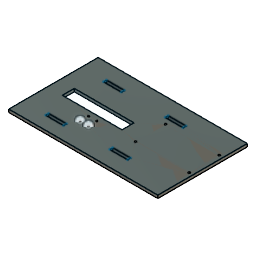
CAD for mechanical car (Autodesk Fusion 360 archive; units mm, degrees)
design "Main Body"
part number: 2026-02-16-11-50-54-130
Autodesk Fusion 360 part; units mm, degrees
(part 1 of 14)
sketch "Sketch1" plane through (0, 0, 0) normal (0, 0, 1) x (1, 0, 0)
  line L0 (0, 0) -> (250, 0)
  line L1 (250, 0) -> (250, 150)
  line L2 (250, 150) -> (0, 150)
  line L3 (0, 150) -> (0, 0)
  line L4 (25, 65) -> (25, 85)
  line L5 (25, 85) -> (125, 85)
  line L6 (125, 85) -> (125, 65)
  line L7 (125, 65) -> (25, 65)
  dimension "d1" = 250
  dimension "d2" = 150
  dimension "d5" = 100
  dimension "d42" = 20
  constraint horizontal L0
  constraint vertical L1
  constraint horizontal L2
  constraint vertical L3
  constraint coincident L0.start L3.end
  constraint perpendicular L5 L6
  constraint perpendicular L4 L7
  measures "d1" distance of L0.start L0.end
  measures "d2" distance of L0.start L2.end
  measures "d5" distance of L4.end L5.end
  measures "d42" distance of L5.end L6.end
extrude "Extrude1" add sketch "Sketch1" along normal blind 5
sketch "Sketch2" plane through (0, 0, 5) normal (0, 0, 1) x (-1, 0, 0)
  line L0 (-125, -85) -> (-125, -65)
  line L1 (-125, -65) -> (-25, -65)
  line L2 (-25, -65) -> (-25, -85)
  line L3 (-25, -85) -> (-125, -85)
  line L4 (0, -150) -> (0, 0)
  line L5 (0, 0) -> (-250, 0)
  line L6 (-250, 0) -> (-250, -150)
  line L7 (-250, -150) -> (0, -150)
  line L8 (-40, -22) -> (-70, -22)
  line L9 (-40, -27) -> (-70, -27)
  line L10 (-70, -27) -> (-70, -22)
  line L11 (-40, -22) -> (-40, -27)
  line L12 (-40, -124) -> (-40, -119)
  line L13 (-40, -124) -> (-70, -124)
  line L14 (-70, -119) -> (-70, -124)
  line L15 (-40, -119) -> (-70, -119)
  line L16 (-143.376, -31) -> (-143.376, -26)
  line L17 (-173.376, -26) -> (-143.376, -26)
  line L18 (-173.376, -26) -> (-173.376, -31)
  line L19 (-173.376, -31) -> (-143.376, -31)
  line L20 (-173.376, -124) -> (-173.376, -119)
  line L21 (-173.376, -119) -> (-143.376, -119)
  line L22 (-143.376, -119) -> (-143.376, -124)
  line L23 (-173.376, -124) -> (-143.376, -124)
  dimension "d10" = 30
  dimension "d34" = 26
  dimension "d35" = 5
  dimension "d36" = 26
  dimension "d37" = 5
  dimension "d38" = 26
  dimension "d39" = 5
  dimension "d40" = 5
  dimension "d41" = 22
  constraint perpendicular L8 L10
  constraint perpendicular L9 L11
  measures "d10" distance of L8.start L8.end
  measures "d34" distance of L7 L13
  measures "d35" distance of L13 L15
  measures "d36" distance of L7 L23
  measures "d37" distance of L21 L23
  measures "d38" distance of L5 L17
  measures "d39" distance of L17 L19
  measures "d40" distance of L8 L9
  measures "d41" distance of L5 L8
extrude "Extrude2" cut sketch "Sketch2" against normal blind 10 contours L8 L9 L10 L11 | L12 L13 L14 L15 | L16 L17 L18 L19 | L20 L21 L22 L23
sketch "Sketch3" plane through (0, 0, 5) normal (0, 0, 1) x (-1, 0, 0)
  line L0 (-143.376, -31) -> (-173.376, -31)
  line L1 (-173.376, -31) -> (-173.376, -26)
  line L2 (-173.376, -26) -> (-143.376, -26)
  line L3 (-143.376, -26) -> (-143.376, -31)
  line L4 (-143.376, -124) -> (-173.376, -124)
  line L5 (-173.376, -124) -> (-173.376, -119)
  line L6 (-173.376, -119) -> (-143.376, -119)
  line L7 (-143.376, -119) -> (-143.376, -124)
  line L8 (-70, -27) -> (-70, -22)
  line L9 (-70, -22) -> (-40, -22)
  line L10 (-40, -22) -> (-40, -27)
  line L11 (-40, -27) -> (-70, -27)
  line L12 (-70, -119) -> (-40, -119)
  line L13 (-40, -119) -> (-40, -124)
  line L14 (-40, -124) -> (-70, -124)
  line L15 (-70, -124) -> (-70, -119)
  line L16 (-125, -85) -> (-125, -65)
  line L17 (-125, -65) -> (-25, -65)
  line L18 (-25, -65) -> (-25, -85)
  line L19 (-25, -85) -> (-125, -85)
  line L20 (0, -150) -> (0, 0)
  line L21 (0, 0) -> (-250, 0)
  line L22 (-250, 0) -> (-250, -150)
  line L23 (-250, -150) -> (0, -150)
  circle A0 centre (-91.302, -56.5) radius 1.75
  circle A1 centre (-91.302, -42.5) radius 1.75
  circle A2 centre (-77.302, -56.5) radius 1.75
  circle A3 centre (-77.302, -42.5) radius 1.75
  line L24 (-245.676, -150) -> (-245.676, -100) construction
  line L25 (-245.676, 0) -> (-245.676, -50) construction
  point P0 (-245.676, -100)
  point P1 (-245.676, -50)
  dimension "d21" = 3.5
  dimension "d43" = 4.324
  dimension "d44" = 4.324
  constraint coincident L23 L24.start
  constraint perpendicular L23 L24
  constraint coincident L21 L25.start
  constraint perpendicular L21 L25
  constraint coincident P0 L24.end
  constraint coincident P1 L25.end
  measures "d21" diameter of A0
  measures "d43" distance of L22 L24
  measures "d44" distance of L22 L25
extrude "Extrude3" cut sketch "Sketch3" against normal blind 5 contours A0 | A1 | A2 | A3
thread "Thread1" "ISO Metric profile 3.5 M3.5x0.6 M3.5x0.6 6H" major diameter 3.5995 minor diameter 2.93 pitch 0.6 angle 60 resizes the face on face at (75.6894, 57.1798, 3.3333)
thread "Thread2" "ISO Metric profile 3.5 M3.5x0.6 M3.5x0.6 6H" major diameter 3.5995 minor diameter 2.93 pitch 0.6 angle 60 resizes the face on face at (89.6894, 57.1798, 3.3333)
thread "Thread3" "ISO Metric profile 3.5 M3.5x0.6 M3.5x0.6 6H" major diameter 3.5995 minor diameter 2.93 pitch 0.6 angle 60 resizes the face on face at (75.6894, 43.1798, 3.3333)
thread "Thread4" "ISO Metric profile 3.5 M3.5x0.6 M3.5x0.6 6H" major diameter 3.5995 minor diameter 2.93 pitch 0.6 angle 60 resizes the face on face at (89.6894, 43.1798, 3.3333)
sketch "Sketch4" plane through (0, 0, 5) normal (0, 0, 1) x (-1, 0, 0)
  circle A0 centre (-91.302, -56.5) radius 1.465
  circle A1 centre (-91.302, -42.5) radius 1.465
  circle A2 centre (-77.302, -56.5) radius 1.465
  circle A3 centre (-77.302, -42.5) radius 1.465
  line L0 (-143.376, -31) -> (-173.376, -31)
  line L1 (-173.376, -31) -> (-173.376, -26)
  line L2 (-173.376, -26) -> (-143.376, -26)
  line L3 (-143.376, -26) -> (-143.376, -31)
  line L4 (-143.376, -124) -> (-173.376, -124)
  line L5 (-173.376, -124) -> (-173.376, -119)
  line L6 (-173.376, -119) -> (-143.376, -119)
  line L7 (-143.376, -119) -> (-143.376, -124)
  line L8 (-70, -27) -> (-70, -22)
  line L9 (-70, -22) -> (-40, -22)
  line L10 (-40, -22) -> (-40, -27)
  line L11 (-40, -27) -> (-70, -27)
  line L12 (-70, -119) -> (-40, -119)
  line L13 (-40, -119) -> (-40, -124)
  line L14 (-40, -124) -> (-70, -124)
  line L15 (-70, -124) -> (-70, -119)
  line L16 (-125, -85) -> (-125, -65)
  line L17 (-125, -65) -> (-25, -65)
  line L18 (-25, -65) -> (-25, -85)
  line L19 (-25, -85) -> (-125, -85)
  line L20 (0, -150) -> (0, 0)
  line L21 (0, 0) -> (-250, 0)
  line L22 (-250, 0) -> (-250, -150)
  line L23 (-250, -150) -> (0, -150)
sketch "Sketch5" plane through (0, 0, 5) normal (0, 0, 1) x (-1, 0, 0)
  circle A0 centre (-91.302, -56.5) radius 1.465
  circle A1 centre (-91.302, -42.5) radius 1.465
  circle A2 centre (-77.302, -56.5) radius 1.465
  circle A3 centre (-77.302, -42.5) radius 1.465
  line L0 (-143.376, -31) -> (-173.376, -31)
  line L1 (-173.376, -31) -> (-173.376, -26)
  line L2 (-173.376, -26) -> (-143.376, -26)
  line L3 (-143.376, -26) -> (-143.376, -31)
  line L4 (-143.376, -124) -> (-173.376, -124)
  line L5 (-173.376, -124) -> (-173.376, -119)
  line L6 (-173.376, -119) -> (-143.376, -119)
  line L7 (-143.376, -119) -> (-143.376, -124)
  line L8 (-70, -27) -> (-70, -22)
  line L9 (-70, -22) -> (-40, -22)
  line L10 (-40, -22) -> (-40, -27)
  line L11 (-40, -27) -> (-70, -27)
  line L12 (-70, -119) -> (-40, -119)
  line L13 (-40, -119) -> (-40, -124)
  line L14 (-40, -124) -> (-70, -124)
  line L15 (-70, -124) -> (-70, -119)
  line L16 (-125, -85) -> (-125, -65)
  line L17 (-125, -65) -> (-25, -65)
  line L18 (-25, -65) -> (-25, -85)
  line L19 (-25, -85) -> (-125, -85)
  line L20 (0, -150) -> (0, 0)
  line L21 (0, 0) -> (-250, 0)
  line L22 (-250, 0) -> (-250, -150)
  line L23 (-250, -150) -> (0, -150)
  line L24 (-244.9961, -70.043) -> (-245.7331, -70.043) construction
  line L25 (-245.7331, -70.043) -> (-240.4599, -70.043) construction
  circle A4 centre (-243.5877, -109.541) radius 2
  circle A5 centre (-153.5877, -109.541) radius 2
  line L26 (-153.5877, -119) -> (-153.5877, -109.541)
  line L27 (-153.5877, -109.541) -> (-243.5877, -109.541)
  line L28 (-153.5802, -70.983) -> (-153.5877, -59.041)
  circle A6 centre (-153.5877, -59.041) radius 2
  line L29 (-153.5877, -59.041) -> (-243.5877, -59.0974)
  circle A7 centre (-243.5877, -59.0974) radius 2
  line L30 (-153.5877, -109.541) -> (-153.5877, -59.041)
  point P0 (-243.5877, -109.541)
  point P1 (-153.5877, -109.541)
  dimension "d46" = 4
  dimension "d47" = 4
  dimension "d52" = 9.459
  dimension "d53" = 90
  dimension "d56" = 11.942
  dimension "d57" = 4
  dimension "d58" = 90
  dimension "d59" = 4
  dimension "d62" = 50.5
  constraint coincident P0 A4.centre
  constraint coincident P1 A5.centre
  constraint coincident L6 L26.start
  constraint perpendicular L6 L26
  constraint perpendicular L26 L27
  constraint coincident L28.end A6.centre
  constraint perpendicular L28 L29
  constraint coincident L29.end A7.centre
  constraint perpendicular L27 L30
  measures "d46" diameter of A4
  measures "d47" diameter of A5
  measures "d52" distance of L26.start P1
  measures "d53" distance of P1 P0
  measures "d56" distance of L28.start L28.end
  measures "d57" diameter of A6
  measures "d58" distance of L28.end L29.end
  measures "d59" diameter of A7
  measures "d62" distance of P1 L28.end
hole "Hole1" at (243.5877, 109.541, 5) at (153.5877, 109.541, 5) at (153.5877, 59.041, 5) at (243.5877, 59.0974, 5) direction (0, 0, -1) diameter 3.332 depth 15 tip angle 180
thread "Thread5" "ISO Metric profile 4.0 M4x0.7 M4x0.7 6H" major diameter 4.1095 minor diameter 3.332 pitch 0.7 angle 60 resizes the face on face at (152.5818, 108.213, 3.3333) on face at (242.5818, 57.7694, 3.3333) on face at (242.5818, 108.213, 3.3333) on face at (152.5818, 57.713, 3.3333)
sketch "Sketch6" plane through (0, 0, 5) normal (0, 0, 1) x (-1, 0, 0)
  point P0 (-77.3, -42.5)
  point P1 (-91.3, -42.5)
equation "d43 = 2.9 mm + 1.424 mm"
equation "d44 = 2.9 mm + 1.424 mm"

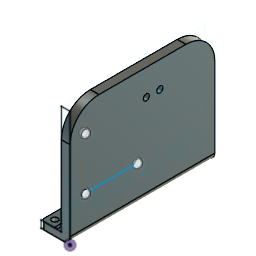
design "bracket left stopping mechanism"
part number: 2026-03-17-00-30-14-356
Autodesk Fusion 360 part; units mm, degrees
sketch "Sketch1" plane through (0, 0, 0) normal (0, 1, 0) x (1, 0, 0)
  line L0 (-20, 0) -> (0, 0)
  line L1 (0, 0) -> (0, -80)
  line L2 (0, -80) -> (-6, -80)
  line L3 (-6, -80) -> (-6, -5)
  line L4 (-6, -5) -> (-20, -5)
  line L5 (-20, -5) -> (-20, 0)
  dimension "d6" = 80
  dimension "d7" = 6
  dimension "d8" = 75
  dimension "d41" = 5
  dimension "d42" = 14
  constraint coincident L0.end L1.start
  constraint horizontal L0
  constraint perpendicular L0 L1
  constraint perpendicular L1 L2
  constraint perpendicular L0 L3
  constraint perpendicular L3 L4
  constraint perpendicular L0 L5
  measures "d6" distance of L0.end L1.end
  measures "d7" distance of L1.end L2.end
  measures "d8" distance of L2.end L3.end
  measures "d41" distance of L0.start L4.end
  measures "d42" distance of L3.end L4.end
extrude "Extrude1" add sketch "Sketch1" along normal blind 100
sketch "Sketch2" plane through (-6, 0, 0) normal (-1, 0, 0) x (0, -1, 0)
  line L0 (0, 5) -> (0, 80)
  line L1 (0, 80) -> (-100, 80)
  line L2 (-100, 80) -> (-100, 5)
  line L3 (-100, 5) -> (0, 5)
sketch "Sketch3" plane through (-6, 0, 0) normal (-1, 0, 0) x (0, -1, 0)
  circle A0 centre (-62, 62) radius 2.1
  line L0 (0, 80) -> (-100, 80)
  line L1 (0, 5) -> (-100, 5)
  line L2 (0, 5) -> (0, 80)
  line L3 (0, 0) -> (0, 80)
  dimension "d12" = 4.2
  dimension "d57" = 62
  measures "d12" diameter of A0
  measures "d57" distance of A0.centre L3
sketch "Sketch4" plane through (-6, 0, 0) normal (-1, 0, 0) x (0, -1, 0)
sketch "Sketch5" plane through (-6, 0, 0) normal (-1, 0, 0) x (0, -1, 0)
extrude "Extrude2" cut sketch "Sketch3" against normal blind 6
fillet "Fillet1" radius 20 1 edges at (-3, 100, 80)
fillet "Fillet2" radius 20 1 edges at (-3, 0, 80)
fillet "Fillet3" radius 5 1 edges at (-6, 50, 5)
sketch "Sketch7" plane through (0, 0, 5) normal (0, 0, 1) x (-1, 0, 0)
  line L0 (11, 0) -> (11, -100)
  line L1 (11, -100) -> (20, -100)
  line L2 (20, -100) -> (20, 0)
  line L3 (20, 0) -> (11, 0)
sketch "Sketch8" plane through (0, 0, 5) normal (0, 0, 1) x (-1, 0, 0)
  circle A0 centre (15.5, -5) radius 2.1
  dimension "d28" = 4.2
  measures "d28" diameter of A0
extrude "Extrude4" cut sketch "Sketch8" against normal blind 5
sketch "Sketch9" plane through (0, 0, 5) normal (0, 0, 1) x (-1, 0, 0)
sketch "Sketch10" plane through (0, 0, 5) normal (0, 0, 1) x (-1, 0, 0)
  circle A0 centre (15, -95) radius 2.1
  dimension "d32" = 4.2
  measures "d32" diameter of A0
extrude "Extrude5" cut sketch "Sketch10" against normal blind 5
fillet "Fillet4" radius 2 1 edges at (-20, 0, 2.5)
fillet "Fillet5" radius 2 1 edges at (-20, 100, 2.5)
fillet "Fillet6" radius 5 1 edges at (0, 50, 0)
sketch "Sketch11" plane through (0, 0, 0) normal (1, 0, 0) x (0, 1, 0)
  line L0 (0, 5) -> (100, 5)
  line L1 (100, 5) -> (100, 60)
  arc A0 (100, 60) -> (80, 80) centre (80, 60) ccw
  line L2 (80, 80) -> (20, 80)
  arc A1 (20, 80) -> (0, 60) centre (20, 60) ccw
  line L3 (0, 60) -> (0, 5)
  circle A2 centre (62, 62) radius 2.1
sketch "Sketch12" plane through (0, 0, 0) normal (1, 0, 0) x (0, 1, 0)
sketch "Sketch13" plane through (0, 0, 0) normal (1, 0, 0) x (0, 1, 0)
sketch "Sketch14" plane through (0, 0, 0) normal (1, 0, 0) x (0, 1, 0)
sketch "Sketch15" plane through (0, 0, 0) normal (1, 0, 0) x (0, 1, 0)
sketch "Sketch17" plane through (0, 0, 0) normal (1, 0, 0) x (0, 1, 0)
  circle A0 centre (10, 62) radius 2.1
  dimension "d54" = 4.2
  measures "d54" diameter of A0
extrude "Extrude6" cut sketch "Sketch17" against normal blind 6
sketch "Sketch18" plane through (0, 0, 0) normal (1, 0, 0) x (0, 1, 0)
sketch "Sketch19" plane through (0, 0, 0) normal (1, 0, 0) x (0, 1, 0)
sketch "Sketch20" plane through (0, 0, 0) normal (1, 0, 0) x (0, 1, 0)
  circle A0 centre (10, 26) radius 2.1
  dimension "d59" = 4.2
  measures "d59" diameter of A0
extrude "Extrude7" cut sketch "Sketch20" against normal blind 6
sketch "Sketch21" plane through (0, 0, 0) normal (1, 0, 0) x (0, 1, 0)
sketch "Sketch22" plane through (0, 0, 0) normal (1, 0, 0) x (0, 1, 0)
  point P0 (10, 62)
sketch "Sketch23" plane through (0, 0, 0) normal (1, 0, 0) x (0, 1, 0)
sketch "Sketch24" plane through (0, 0, 0) normal (1, 0, 0) x (0, 1, 0)
  line L0 (10, 26) -> (46, 26)
  dimension "d62" = 36
  constraint horizontal L0
  measures "d62" distance of L0.start L0.end
sketch "Sketch25" plane through (0, 0, 0) normal (1, 0, 0) x (0, 1, 0)
  line L0 (10, 62) -> (52.686, 62)
  circle A0 centre (52.686, 62) radius 2.1
  dimension "d63" = 42.686
  dimension "d64" = 4.2
  constraint horizontal L0
  constraint coincident L0.end A0.centre
  measures "d63" distance of L0.start L0.end
  measures "d64" diameter of A0
extrude "Extrude8" cut sketch "Sketch25" against normal blind 6

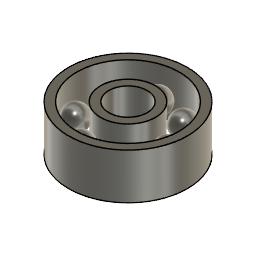
design "Bearing 4.2x13"
part number: 2026-09-12-01-25-43-170
Autodesk Fusion 360 part; units mm, degrees
sketch "Sketch1" plane through (0, 0, 0) normal (0, 1, 0) x (1, 0, 0)
  line L0 (2.1, -2.5) -> (3, -2.5)
  line L1 (3, -2.5) -> (3, 2.5)
  line L2 (3, 2.5) -> (2.1, 2.5)
  line L3 (2.1, 2.5) -> (2.1, -2.5)
  line L4 (5.6, -2.5) -> (6.5, -2.5)
  line L5 (6.5, -2.5) -> (6.5, 2.5)
  line L6 (6.5, 2.5) -> (5.6, 2.5)
  line L7 (5.6, 2.5) -> (5.6, -2.5)
  line L8 (0, -10) -> (0, 10) construction
revolve "Revolve1" add sketch "Sketch1" angle 360 about axis through (0, 0, 10) along (0, 0, -1) contours L0 L1 L2 L3 makes body 1
revolve "Revolve2" add sketch "Sketch1" angle 360 about axis through (0, 0, 10) along (0, 0, -1) separate body contours L4 L5 L6 L7 makes body 2
sketch "Sketch2" plane through (0, 0, 0) normal (0, 1, 0) x (1, 0, 0)
  line L0 (4.3, -10) -> (4.3, 10) construction
  arc A0 (4.3, -1.3) -> (4.3, 1.3) centre (4.3, 0) ccw
  line L1 (4.3, 1.3) -> (4.3, -1.3)
revolve "Revolve3" add sketch "Sketch2" angle 360 about axis through (4.3, 0, 10) along (0, 0, -1) separate body makes body 3
pattern_circular "C-Pattern2" count 7 over 360 about axis through (0, 0, 1.75) along (0, 0, 1) of bodies 3 makes body 4 at (3.6897, 4.1339, 0.2766) makes body 5 at (-0.9315, 5.4622, 0.2766) makes body 6 at (-4.8513, 2.6773, 0.2766) makes body 7 at (-5.1179, -2.1236, 0.2766) makes body 8 at (-1.5307, -5.3254, 0.2766) makes body 9 at (3.2092, -4.5171, 0.2766)
named bodies: "Inner Race", "Outer Race", "Ball", "Ball (1)", "Ball (2)", "Ball (3)", "Ball (4)", "Ball (5)", "Ball (6)"

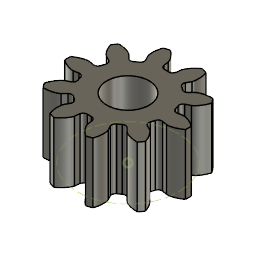
design "Smaller 10 Tooth Gear"
description: Spur Gear; Module: 1.0; Num Teeth: 10; Pressure Angle: 20.0; Backlash: 0.00 mm
part number: 2026-09-03-00-38-16-628
Autodesk Fusion 360 part; units mm, degrees
sketch "Base Circle" plane through (0, 0, 0) normal (0, 0, 1) x (1, 0, 0)
  circle A0 centre (0, 0) radius 3.843
  circle A1 centre (0, 0) radius 2.1
extrude "Extrude1" add sketch "Base Circle" along normal blind 6
sketch "Gear Tooth" plane through (0, 0, 0) normal (0, 0, 1) x (1, 0, 0)
  spline S0 degree 5 poles (4.6291, -0.8041) (4.6329, -0.8047) (4.6405, -0.8059) (4.6519, -0.8073) (4.6672, -0.8084) (4.6864, -0.8088) (4.7057, -0.8085) (4.7251, -0.8077) (4.7445, -0.8066) (4.7639, -0.8054) (4.7834, -0.804) (4.8029, -0.8024) (4.8224, -0.8004) (4.842, -0.7981) (4.8616, -0.7955) (4.8812, -0.7924) (4.9009, -0.7891) (4.9205, -0.7856) (4.9402, -0.7818) (4.9599, -0.7778) (4.9796, -0.7737) (4.9993, -0.7693) (5.019, -0.7646) (5.0388, -0.7598) (5.0585, -0.7547) (5.0783, -0.7493) (5.098, -0.7438) (5.1178, -0.738) (5.1375, -0.7321) (5.1573, -0.7259) (5.177, -0.7196) (5.1968, -0.7131) (5.2165, -0.7063) (5.2363, -0.6994) (5.256, -0.6923) (5.2757, -0.685) (5.2955, -0.6775) (5.3152, -0.6698) (5.3349, -0.6619) (5.3546, -0.6538) (5.3743, -0.6456) (5.394, -0.6372) (5.4136, -0.6286) (5.4333, -0.6198) (5.4529, -0.6109) (5.4725, -0.6018) (5.4921, -0.5925) (5.5117, -0.583) (5.5312, -0.5734) (5.5508, -0.5636) (5.5703, -0.5536) (5.5898, -0.5435) (5.6093, -0.5332) (5.6287, -0.5228) (5.6482, -0.5121) (5.6676, -0.5013) (5.6869, -0.4904) (5.7063, -0.4793) (5.7256, -0.468) (5.7449, -0.4566) (5.7642, -0.445) (5.7834, -0.4332) (5.8026, -0.4213) (5.8218, -0.4093) (5.8409, -0.397) (5.86, -0.3847) (5.8791, -0.3721) (5.8982, -0.3595) (5.9172, -0.3466) (5.9361, -0.3336) (5.9551, -0.3205) (5.9702, -0.3099) (5.9815, -0.3018) (5.989, -0.2964) (5.9928, -0.2937) knots 0 0 0 0 0 0 0.01428571 0.02857143 0.04285714 0.05714286 0.07142857 0.08571429 0.1 0.11428571 0.12857143 0.14285714 0.15714286 0.17142857 0.18571429 0.2 0.21428571 0.22857143 0.24285714 0.25714286 0.27142857 0.28571429 0.3 0.31428571 0.32857143 0.34285714 0.35714286 0.37142857 0.38571429 0.4 0.41428571 0.42857143 0.44285714 0.45714286 0.47142857 0.48571429 0.5 0.51428571 0.52857143 0.54285714 0.55714286 0.57142857 0.58571429 0.6 0.61428571 0.62857143 0.64285714 0.65714286 0.67142857 0.68571429 0.7 0.71428571 0.72857143 0.74285714 0.75714286 0.77142857 0.78571429 0.8 0.81428571 0.82857143 0.84285714 0.85714286 0.87142857 0.88571429 0.9 0.91428571 0.92857143 0.94285714 0.95714286 0.97142857 0.98571429 1 1 1 1 1 1
  spline S1 degree 5 poles (4.6291, 0.8041) (4.6329, 0.8047) (4.6405, 0.8059) (4.6519, 0.8073) (4.6672, 0.8084) (4.6864, 0.8088) (4.7057, 0.8085) (4.7251, 0.8077) (4.7445, 0.8066) (4.7639, 0.8054) (4.7834, 0.804) (4.8029, 0.8024) (4.8224, 0.8004) (4.842, 0.7981) (4.8616, 0.7955) (4.8812, 0.7924) (4.9009, 0.7891) (4.9205, 0.7856) (4.9402, 0.7818) (4.9599, 0.7778) (4.9796, 0.7737) (4.9993, 0.7693) (5.019, 0.7646) (5.0388, 0.7598) (5.0585, 0.7547) (5.0783, 0.7493) (5.098, 0.7438) (5.1178, 0.738) (5.1375, 0.7321) (5.1573, 0.7259) (5.177, 0.7196) (5.1968, 0.7131) (5.2165, 0.7063) (5.2363, 0.6994) (5.256, 0.6923) (5.2757, 0.685) (5.2955, 0.6775) (5.3152, 0.6698) (5.3349, 0.6619) (5.3546, 0.6538) (5.3743, 0.6456) (5.394, 0.6372) (5.4136, 0.6286) (5.4333, 0.6198) (5.4529, 0.6109) (5.4725, 0.6018) (5.4921, 0.5925) (5.5117, 0.583) (5.5312, 0.5734) (5.5508, 0.5636) (5.5703, 0.5536) (5.5898, 0.5435) (5.6093, 0.5332) (5.6287, 0.5228) (5.6482, 0.5121) (5.6676, 0.5013) (5.6869, 0.4904) (5.7063, 0.4793) (5.7256, 0.468) (5.7449, 0.4566) (5.7642, 0.445) (5.7834, 0.4332) (5.8026, 0.4213) (5.8218, 0.4093) (5.8409, 0.397) (5.86, 0.3847) (5.8791, 0.3721) (5.8982, 0.3595) (5.9172, 0.3466) (5.9361, 0.3336) (5.9551, 0.3205) (5.9702, 0.3099) (5.9815, 0.3018) (5.989, 0.2964) (5.9928, 0.2937) knots 0 0 0 0 0 0 0.01428571 0.02857143 0.04285714 0.05714286 0.07142857 0.08571429 0.1 0.11428571 0.12857143 0.14285714 0.15714286 0.17142857 0.18571429 0.2 0.21428571 0.22857143 0.24285714 0.25714286 0.27142857 0.28571429 0.3 0.31428571 0.32857143 0.34285714 0.35714286 0.37142857 0.38571429 0.4 0.41428571 0.42857143 0.44285714 0.45714286 0.47142857 0.48571429 0.5 0.51428571 0.52857143 0.54285714 0.55714286 0.57142857 0.58571429 0.6 0.61428571 0.62857143 0.64285714 0.65714286 0.67142857 0.68571429 0.7 0.71428571 0.72857143 0.74285714 0.75714286 0.77142857 0.78571429 0.8 0.81428571 0.82857143 0.84285714 0.85714286 0.87142857 0.88571429 0.9 0.91428571 0.92857143 0.94285714 0.95714286 0.97142857 0.98571429 1 1 1 1 1 1
  arc A0 (5.9928, -0.2937) -> (5.9928, 0.2937) centre (0, 0) ccw
  line L0 (3.7765, -0.656) -> (4.6291, -0.8041)
  line L1 (3.7765, 0.656) -> (4.6291, 0.8041)
  line L2 (3.7765, -0.656) -> (3.7765, 0.656)
  point P0 (4.7229, -0.8077)
  point P1 (4.8183, -0.8008)
  point P2 (4.9148, -0.7866)
  point P3 (5.0121, -0.7662)
  point P4 (5.11, -0.7403)
  point P5 (5.2082, -0.7091)
  point P6 (5.3067, -0.673)
  point P7 (5.4054, -0.6322)
  point P8 (5.504, -0.5867)
  point P9 (5.6025, -0.5368)
  point P10 (5.7007, -0.4824)
  point P11 (5.7986, -0.4238)
  point P12 (5.896, -0.3609)
  point P13 (4.7229, 0.8077)
  point P14 (4.8183, 0.8008)
  point P15 (4.9148, 0.7866)
  point P16 (5.0121, 0.7662)
  point P17 (5.11, 0.7403)
  point P18 (5.2082, 0.7091)
  point P19 (5.3067, 0.673)
  point P20 (5.4054, 0.6322)
  point P21 (5.504, 0.5867)
  point P22 (5.6025, 0.5368)
  point P23 (5.7007, 0.4824)
  point P24 (5.7986, 0.4238)
  point P25 (5.896, 0.3609)
extrude "Extrude2" add sketch "Gear Tooth" along normal blind 6
fillet "Fillet1" radius 0.38 2 edges at (3.7863, -0.6577, 3) (3.7863, 0.6577, 3)
pattern_circular "C-Pattern1" count 10 over 360 about axis through (0, 0, 0) along (0, 0, 1) of "Extrude2", "Fillet1"
sketch "Diametrial Pitch Circle" plane through (0, 0, 0) normal (0, 0, 1) x (1, 0, 0)
  circle A0 centre (0, 0) radius 5 construction
named bodies: "Spur Gear (10 teeth)"

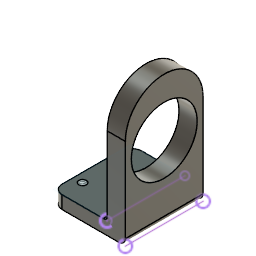
design "motor mount"
part number: 2026-09-09-23-18-51-643
Autodesk Fusion 360 part; units mm, degrees
sketch "Sketch1" plane through (0, 0, 0) normal (0, 1, 0) x (1, 0, 0)
  line L0 (0, 0) -> (0, -50)
  line L1 (0, -50) -> (-7.035, -50)
  line L2 (-7.035, -50) -> (-7.035, -5)
  line L3 (-7.035, -5) -> (-27.965, -5)
  line L4 (-27.965, -5) -> (-27.965, 0)
  line L5 (-27.965, 0) -> (0, 0)
  dimension "d1" = 50
  dimension "d2" = 7.035
  dimension "d3" = 45
  dimension "d4" = 20.93
  constraint coincident L0.start L5.end
  constraint vertical L0
  constraint perpendicular L0 L1
  constraint perpendicular L1 L2
  constraint perpendicular L2 L3
  constraint perpendicular L3 L4
  constraint perpendicular L0 L5
  measures "d1" distance of L0.start L0.end
  measures "d2" distance of L0.end L1.end
  measures "d3" distance of L1.end L2.end
  measures "d4" distance of L2.end L3.end
extrude "Extrude1" add sketch "Sketch1" along normal blind 30
sketch "Sketch2" plane through (0, 0, 0) normal (1, 0, 0) x (0, 1, 0)
sketch "Sketch4" plane through (0, 0, 0) normal (1, 0, 0) x (0, 1, 0)
  line L0 (0, 0) -> (30, 0)
  dimension "d9" = 30
  measures "d9" distance of L0.start L0.end
sketch "Sketch5" plane through (0, 0, 0) normal (1, 0, 0) x (0, 1, 0)
sketch "Sketch6" plane through (0, 0, 0) normal (1, 0, 0) x (0, 1, 0)
fillet "Fillet3" radius 2.5 1 edges at (0, 15, 0)
sketch "Sketch8" plane through (0, 0, 5) normal (0, 0, 1) x (-1, 0, 0)
  line L0 (27.965, 0) -> (7.035, 0)
  line L1 (7.035, 0) -> (7.035, -30)
  line L2 (7.035, -30) -> (27.965, -30)
  line L3 (27.965, -30) -> (27.965, 0)
sketch "Sketch9" plane through (0, 0, 5) normal (0, 0, 1) x (-1, 0, 0)
  circle A0 centre (10.4981, -26.535) radius 1.465
  line L0 (7.035, -30) -> (27.965, -30)
  dimension "d20" = 2.93
  dimension "d24" = 3.465
  measures "d20" diameter of A0
  measures "d24" distance of A0.centre L0
sketch "Sketch10" plane through (0, 0, 5) normal (0, 0, 1) x (1, 0, 0)
sketch "Sketch11" plane through (0, 0, 5) normal (0, 0, 1) x (1, 0, 0)
sketch "Sketch12" plane through (0, 0, 5) normal (0, 0, 1) x (-1, 0, 0)
sketch "Sketch13" plane through (0, 0, 5) normal (0, 0, 1) x (-1, 0, 0)
sketch "Sketch14" plane through (0, 0, 5) normal (0, 0, 1) x (-1, 0, 0)
  line L0 (7.035, 0) -> (7.035, -30)
sketch "Sketch21" plane through (0, 0, 5) normal (0, 0, 1) x (-1, 0, 0)
sketch "Sketch22" plane through (0, 0, 5) normal (0, 0, 1) x (-1, 0, 0)
sketch "Sketch23" plane through (0, 0, 5) normal (0, 0, 1) x (-1, 0, 0)
sketch "Sketch25" plane through (0, 0, 5) normal (0, 0, 1) x (-1, 0, 0)
fillet "Fillet4" radius 4.5 1 edges at (-27.965, 30, 2.5)
fillet "Fillet5" radius 3.5 1 edges at (-27.965, 0, 2.5)
fillet "Fillet6" radius 1.5 tangency weight 1.75178 1 edges at (-7.035, 15, 5)
sketch "Sketch32" plane through (0, 0, 5) normal (0, 0, 1) x (-1, 0, 0)
sketch "Sketch33" plane through (0, 0, 5) normal (0, 0, 1) x (1, 0, 0)
sketch "Sketch40" plane through (0, 0, 5) normal (0, 0, 1) x (-1, 0, 0)
sketch "Sketch44" plane through (0, 0, 5) normal (0, 0, 1) x (-1, 0, 0)
  circle A0 centre (10.5, -8) radius 1.465
  dimension "d82" = 2.93
  measures "d82" diameter of A0
sketch "Sketch46" plane through (0, 0, 5) normal (0, 0, 1) x (-1, 0, 0)
  circle A0 centre (10.5, -22) radius 1.465
  dimension "d84" = 2.93
  measures "d84" diameter of A0
sketch "Sketch48" plane through (0, 0, 5) normal (0, 0, 1) x (-1, 0, 0)
  circle A0 centre (24.5, -22) radius 1.465
  dimension "d86" = 2.93
  measures "d86" diameter of A0
sketch "Sketch49" plane through (0, 0, 5) normal (0, 0, 1) x (-1, 0, 0)
  circle A0 centre (24.5, -8) radius 1.465
  dimension "d87" = 2.93
  measures "d87" diameter of A0
extrude "Extrude8" cut sketch "Sketch49" against normal blind 10
extrude "Extrude9" cut sketch "Sketch44" against normal blind 10
extrude "Extrude10" cut sketch "Sketch46" against normal blind 10
extrude "Extrude11" cut sketch "Sketch48" against normal blind 10
thread "Thread5" "ISO Metric profile 3.5 M3.5x0.6 M3.5x0.6 6H" major diameter 3.5995 minor diameter 2.93 pitch 0.6 angle 60 resizes the face on face at (-25.9577, 8.1459, 3.3333)
thread "Thread6" "ISO Metric profile 3.5 M3.5x0.6 M3.5x0.6 6H" major diameter 3.5995 minor diameter 2.93 pitch 0.6 angle 60 resizes the face on face at (-11.9577, 8.1459, 3.3333)
thread "Thread7" "ISO Metric profile 3.5 M3.5x0.6 M3.5x0.6 6H" major diameter 3.5995 minor diameter 2.93 pitch 0.6 angle 60 resizes the face on face at (-11.9577, 22.1459, 3.3333)
thread "Thread8" "ISO Metric profile 3.5 M3.5x0.6 M3.5x0.6 6H" major diameter 3.5995 minor diameter 2.93 pitch 0.6 angle 60 resizes the face on face at (-25.9577, 22.1459, 3.3333)
sketch "Sketch50" plane through (0, 0, 5) normal (0, 0, 1) x (-1, 0, 0)
sketch "Sketch51" plane through (0, 0, 0) normal (0, 1, 0) x (1, 0, 0)
sketch "Sketch52" plane through (0, 0, 0) normal (0, 0, 1) x (1, 0, 0)
sketch "Sketch55" plane through (0, 0, 0) normal (1, 0, 0) x (0, 1, 0)
  line L0 (0, 2.5) -> (30, 2.5)
  line L1 (30, 2.5) -> (30, 50)
  line L2 (30, 50) -> (0, 50)
  line L3 (0, 50) -> (0, 2.5)
  circle A0 centre (15, 27.9) radius 12.7
  dimension "d106" = 25.4
  measures "d106" diameter of A0
extrude "Extrude12" cut sketch "Sketch55" against normal blind 10 contours A0
fillet "Fillet7" radius 15 1 edges at (-3.5175, 30, 50)
fillet "Fillet8" radius 15 1 edges at (-3.5175, 0, 50)

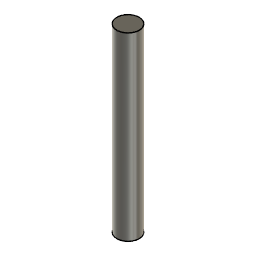
design "bracket shaft"
part number: 2026-03-17-00-51-08-330
Autodesk Fusion 360 part; units mm, degrees
sketch "Sketch1" plane through (0, 0, 0) normal (0, 0, 1) x (1, 0, 0)
cylinder "CylinderPrimitive1" add diameter 4 height 32 placed x (1, 0, 0) y (0, 1, 0) z (0, 0, 1) at (0, 0, 0)
move_body "Move1" bodies 1 to x (1, 0, 0) y (0, 1, 0) z (0, 0, 1) at (0, 0, 11)

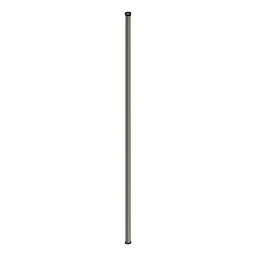
design "Axle"
part number: 2026-03-02-11-54-45-351
Autodesk Fusion 360 part; units mm, degrees
sketch "Sketch1" plane through (0, 0, 0) normal (0, 0, 1) x (1, 0, 0)
  circle A0 centre (0, 0) radius 2
  dimension "d1" = 4
  constraint coincident A0.centre origin
  measures "d1" diameter of A0
extrude "Extrude1" add sketch "Sketch1" along normal blind 190

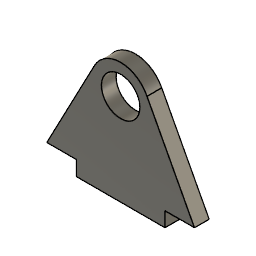
design "Axle Holder"
part number: 2026-02-16-12-04-03-458
Autodesk Fusion 360 part; units mm, degrees
sketch "Sketch1" plane through (0, 0, 0) normal (0, 1, 0) x (1, 0, 0)
  line L0 (0, 0) -> (30, 0)
  line L1 (30, 0) -> (30, -5)
  line L2 (0, 0) -> (0, -5)
  line L3 (0, -5) -> (-10, -5)
  arc A0 (6.0697, -35.5) -> (23.9303, -35.5) centre (15, -31) ccw
  line L4 (30, -5) -> (40, -5)
  line L5 (6.0697, -35.5) -> (-10, -5)
  line L6 (23.9303, -35.5) -> (40, -5)
  dimension "d2" = 10
  dimension "d8" = 5
  dimension "d9" = 31
  dimension "d10" = 10
  dimension "d11" = 10
  dimension "d12" = 5
  dimension "d13" = 30.5
  dimension "d14" = 30.5
  constraint coincident L0.start L2.start
  constraint horizontal L0
  constraint perpendicular L0 L1
  constraint perpendicular L0 L2
  constraint perpendicular L2 L3
  constraint perpendicular L1 L4
  measures "d2" radius of A0
  measures "d8" distance of L0.start L2.end
  measures "d9" distance of L0 A0.centre
  measures "d10" distance of L2.end L3.end
  measures "d11" distance of L1.end L4.end
  measures "d12" distance of L0.end L1.end
  measures "d13" vertical distance of L4.end A0.end
  measures "d14" vertical distance of L3.end A0.start
extrude "Extrude1" add sketch "Sketch1" along normal blind 5
sketch "Sketch2" plane through (0, 0, 0) normal (0, -1, 0) x (1, 0, 0)
  line L0 (0, 5) -> (0, 0)
  line L1 (0, 0) -> (30, 0)
  line L2 (30, 0) -> (30, 5)
  line L3 (30, 5) -> (40, 5)
  arc A0 (23.9303, 35.5) -> (6.0697, 35.5) centre (15, 31) ccw
  line L4 (-10, 5) -> (0, 5)
  circle A1 centre (15, 31) radius 6.5
  line L5 (6.0697, 35.5) -> (-10, 5)
  line L6 (40, 5) -> (23.9303, 35.5)
  dimension "d5" = 13
  constraint concentric A0 A1
  measures "d5" diameter of A1
extrude "Extrude2" cut sketch "Sketch2" against normal blind 5 contours A1

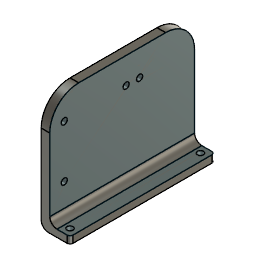
design "Bracket stopping mechanism"
part number: 2026-03-17-00-02-56-113
Autodesk Fusion 360 part; units mm, degrees
sketch "Sketch1" plane through (0, 0, 0) normal (0, 1, 0) x (1, 0, 0)
  line L0 (0, 0) -> (20, 0)
  line L1 (20, 0) -> (20, -5)
  line L2 (20, -5) -> (6, -5)
  line L3 (6, -5) -> (6, -80)
  line L4 (6, -80) -> (0, -80)
  line L5 (0, -80) -> (0, 0)
  dimension "d1" = 20
  dimension "d2" = 5
  dimension "d3" = 14
  dimension "d4" = 75
  dimension "d40" = 80
  dimension "d41" = 6
  constraint coincident L0.start L5.end
  constraint horizontal L0
  constraint perpendicular L0 L1
  constraint perpendicular L1 L2
  constraint perpendicular L2 L3
  constraint perpendicular L3 L4
  constraint perpendicular L0 L5
  measures "d1" distance of L0.start L0.end
  measures "d2" distance of L0.end L1.end
  measures "d3" distance of L1.end L2.end
  measures "d4" distance of L2.end L3.end
  measures "d40" distance of L0.start L4.end
  measures "d41" distance of L3.end L4.end
extrude "Extrude1" add sketch "Sketch1" along normal blind 100
fillet "Fillet1" radius 5 1 edges at (6, 50, 5)
fillet "Fillet2" radius 5 1 edges at (0, 50, 0)
fillet "Fillet3" radius 20 1 edges at (3, 0, 80)
fillet "Fillet4" radius 20 1 edges at (3, 100, 80)
sketch "Sketch2" plane through (6, 0, 0) normal (1, 0, 0) x (0, 1, 0)
  arc A0 (100, 60) -> (80, 80) centre (80, 60) ccw
  line L0 (80, 80) -> (20, 80)
  arc A1 (20, 80) -> (0, 60) centre (20, 60) ccw
  line L1 (0, 60) -> (0, 10)
  line L2 (0, 10) -> (100, 10)
  line L3 (100, 10) -> (100, 60)
sketch "Sketch4" plane through (6, 0, 0) normal (1, 0, 0) x (0, 1, 0)
  circle A0 centre (62, 62) radius 2.1
  line L0 (100, 10) -> (100, 60)
  line L1 (0, 5) -> (100, 5)
  line L2 (0, 60) -> (0, 10)
  dimension "d20" = 4.2
  dimension "d42" = 57
  dimension "d45" = 62
  measures "d20" diameter of A0
  measures "d42" distance of A0.centre L1
  measures "d45" distance of A0.centre L2
extrude "Extrude3" cut sketch "Sketch4" against normal blind 6
sketch "Sketch5" plane through (0, 0, 5) normal (0, 0, 1) x (-1, 0, 0)
  line L0 (-11, -100) -> (-11, 0)
  line L1 (-11, 0) -> (-20, 0)
  line L2 (-20, 0) -> (-20, -100)
  line L3 (-20, -100) -> (-11, -100)
sketch "Sketch6" plane through (0, 0, 5) normal (0, 0, 1) x (-1, 0, 0)
sketch "Sketch7" plane through (0, 0, 5) normal (0, 0, 1) x (-1, 0, 0)
  circle A0 centre (-15, -5) radius 2.1
  circle A1 centre (-15, -95) radius 2.1
  dimension "d27" = 4.2
  dimension "d28" = 4.2
  measures "d27" diameter of A0
  measures "d28" diameter of A1
extrude "Extrude4" cut sketch "Sketch7" against normal blind 5 contours A0
sketch "Sketch8" plane through (0, 0, 5) normal (0, 0, 1) x (-1, 0, 0)
  circle A0 centre (-15, -95) radius 2.1
  dimension "d31" = 4.2
  measures "d31" diameter of A0
extrude "Extrude5" cut sketch "Sketch8" against normal blind 5
fillet "Fillet5" radius 2 1 edges at (20, 100, 2.5)
fillet "Fillet6" radius 2 1 edges at (20, 0, 2.5)
sketch "Sketch9" plane through (6, 0, 0) normal (1, 0, 0) x (0, 1, 0)
sketch "Sketch10" plane through (6, 0, 0) normal (1, 0, 0) x (0, 1, 0)
sketch "Sketch11" plane through (6, 0, 0) normal (1, 0, 0) x (0, 1, 0)
sketch "Sketch12" plane through (6, 0, 0) normal (1, 0, 0) x (0, 1, 0)
sketch "Sketch13" plane through (6, 0, 0) normal (1, 0, 0) x (0, 1, 0)
sketch "Sketch14" plane through (6, 0, 0) normal (1, 0, 0) x (0, 1, 0)
  circle A0 centre (10, 62) radius 2.1
  dimension "d49" = 4.2
  measures "d49" diameter of A0
extrude "Extrude6" cut sketch "Sketch14" against normal blind 6
sketch "Sketch15" plane through (6, 0, 0) normal (1, 0, 0) x (0, 1, 0)
sketch "Sketch16" plane through (6, 0, 0) normal (1, 0, 0) x (0, 1, 0)
  circle A0 centre (10, 26) radius 2.1
  dimension "d54" = 4.2
  measures "d54" diameter of A0
extrude "Extrude7" cut sketch "Sketch16" against normal blind 6
sketch "Sketch17" plane through (6, 0, 0) normal (1, 0, 0) x (0, 1, 0)
  line L0 (10, 62) -> (52.686, 62)
  circle A0 centre (52.686, 62) radius 2.1
  dimension "d57" = 42.686
  dimension "d58" = 4.2
  constraint horizontal L0
  constraint coincident L0.end A0.centre
  measures "d57" distance of L0.start L0.end
  measures "d58" diameter of A0
extrude "Extrude9" cut sketch "Sketch17" against normal blind 6

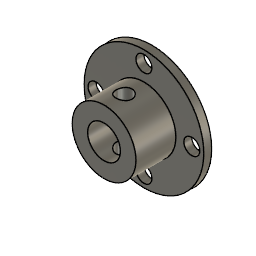
design "Axle Hub"
part number: 2026-02-16-12-21-40-568
Autodesk Fusion 360 part; units mm, degrees
sketch "Sketch1" plane through (0, 0, 0) normal (0, 1, 0) x (1, 0, 0)
  circle A0 centre (0, 0) radius 4
  circle A1 centre (0, 0) radius 2.05
  dimension "d1" = 8
  dimension "d2" = 4.1
  constraint coincident A0.centre A1.centre
  measures "d1" diameter of A0
  measures "d2" diameter of A1
extrude "Extrude1" add sketch "Sketch1" along normal blind 5 makes body 1
sketch "Sketch2" plane through (0, 5, 0) normal (0, 1, 0) x (-1, 0, 0)
  circle A0 centre (0, 0) radius 2.05
  circle A1 centre (0, 0) radius 4
  circle A2 centre (0, 0) radius 7.5
  dimension "d5" = 15
  constraint concentric A0 A2
  measures "d5" diameter of A2
extrude "Extrude2" add sketch "Sketch2" along normal blind 1 separate body contours A2 makes body 2
sketch "Sketch3" plane through (0, 6, 0) normal (0, 1, 0) x (-1, 0, 0)
  circle A0 centre (0, 0) radius 4
  circle A1 centre (0, 0) radius 7.5
  point P0 (0, 6)
  point P1 (0, -6)
  point P2 (-6, 0)
  point P3 (6, 0)
hole "Hole1" at (-6, 6, 0) at (0, 6, -6) at (6, 6, 0) at (0, 6, 6) direction (0, -1, 0) diameter 2 depth 3 tip angle 180 bodies 2
ref_plane "WorkPlane2" through (0, 0, 4) normal (0, 0, 1) x (1, 0, 0)
sketch "Sketch4" plane through (0, 0, 4) normal (0, 0, 1) x (1, 0, 0)
  circle A0 centre (0, 2.5) radius 1
  dimension "d13" = 2.5
  dimension "d14" = 2
  measures "d13" distance of origin A0.centre
  measures "d14" diameter of A0
extrude "Extrude3" cut sketch "Sketch4" against normal blind 9 bodies 1

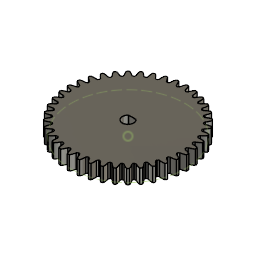
design "Bigger Gear"
description: Spur Gear; Module: 1.0; Num Teeth: 40; Pressure Angle: 20.0; Backlash: 0.00 mm
part number: 2026-02-09-12-07-19-722
Autodesk Fusion 360 part; units mm, degrees
sketch "Base Circle" plane through (0, 0, 0) normal (0, 0, 1) x (1, 0, 0)
  circle A0 centre (0, 0) radius 18.843
  circle A1 centre (0, 0) radius 2
sketch "Gear Tooth" plane through (0, 0, 0) normal (0, 0, 1) x (1, 0, 0)
  spline S0 degree 5 poles (18.7663, -1.0176) (18.7727, -1.0177) (18.7855, -1.0178) (18.8047, -1.0177) (18.8303, -1.0173) (18.8624, -1.0162) (18.8944, -1.0146) (18.9265, -1.0125) (18.9586, -1.0099) (18.9907, -1.0069) (19.0228, -1.0034) (19.0549, -0.9996) (19.087, -0.9955) (19.1191, -0.9911) (19.1512, -0.9864) (19.1833, -0.9815) (19.2154, -0.9763) (19.2475, -0.9708) (19.2796, -0.9651) (19.3117, -0.9591) (19.3438, -0.9529) (19.3759, -0.9464) (19.4079, -0.9398) (19.44, -0.9329) (19.4721, -0.9258) (19.5041, -0.9184) (19.5362, -0.9109) (19.5682, -0.9032) (19.6003, -0.8953) (19.6323, -0.8871) (19.6643, -0.8788) (19.6963, -0.8703) (19.7283, -0.8616) (19.7603, -0.8527) (19.7923, -0.8436) (19.8242, -0.8344) (19.8562, -0.8249) (19.8881, -0.8153) (19.92, -0.8055) (19.952, -0.7956) (19.9839, -0.7855) (20.0158, -0.7752) (20.0476, -0.7647) (20.0795, -0.7541) (20.1114, -0.7433) (20.1432, -0.7324) (20.175, -0.7213) (20.2068, -0.71) (20.2386, -0.6986) (20.2704, -0.687) (20.3022, -0.6753) (20.3339, -0.6634) (20.3656, -0.6513) (20.3974, -0.6392) (20.4291, -0.6268) (20.4607, -0.6143) (20.4924, -0.6017) (20.5241, -0.5889) (20.5557, -0.576) (20.5873, -0.5629) (20.6189, -0.5497) (20.6505, -0.5364) (20.682, -0.5229) (20.7136, -0.5092) (20.7451, -0.4955) (20.7766, -0.4815) (20.8081, -0.4675) (20.8396, -0.4533) (20.871, -0.439) (20.9024, -0.4245) (20.9338, -0.4099) (20.9589, -0.3982) (20.9777, -0.3893) (20.9903, -0.3833) (20.9966, -0.3803) knots 0 0 0 0 0 0 0.01428571 0.02857143 0.04285714 0.05714286 0.07142857 0.08571429 0.1 0.11428571 0.12857143 0.14285714 0.15714286 0.17142857 0.18571429 0.2 0.21428571 0.22857143 0.24285714 0.25714286 0.27142857 0.28571429 0.3 0.31428571 0.32857143 0.34285714 0.35714286 0.37142857 0.38571429 0.4 0.41428571 0.42857143 0.44285714 0.45714286 0.47142857 0.48571429 0.5 0.51428571 0.52857143 0.54285714 0.55714286 0.57142857 0.58571429 0.6 0.61428571 0.62857143 0.64285714 0.65714286 0.67142857 0.68571429 0.7 0.71428571 0.72857143 0.74285714 0.75714286 0.77142857 0.78571429 0.8 0.81428571 0.82857143 0.84285714 0.85714286 0.87142857 0.88571429 0.9 0.91428571 0.92857143 0.94285714 0.95714286 0.97142857 0.98571429 1 1 1 1 1 1
  spline S1 degree 5 poles (18.7663, 1.0176) (18.7727, 1.0177) (18.7855, 1.0178) (18.8047, 1.0177) (18.8303, 1.0173) (18.8624, 1.0162) (18.8944, 1.0146) (18.9265, 1.0125) (18.9586, 1.0099) (18.9907, 1.0069) (19.0228, 1.0034) (19.0549, 0.9996) (19.087, 0.9955) (19.1191, 0.9911) (19.1512, 0.9864) (19.1833, 0.9815) (19.2154, 0.9763) (19.2475, 0.9708) (19.2796, 0.9651) (19.3117, 0.9591) (19.3438, 0.9529) (19.3759, 0.9464) (19.4079, 0.9398) (19.44, 0.9329) (19.4721, 0.9258) (19.5041, 0.9184) (19.5362, 0.9109) (19.5682, 0.9032) (19.6003, 0.8953) (19.6323, 0.8871) (19.6643, 0.8788) (19.6963, 0.8703) (19.7283, 0.8616) (19.7603, 0.8527) (19.7923, 0.8436) (19.8242, 0.8344) (19.8562, 0.8249) (19.8881, 0.8153) (19.92, 0.8055) (19.952, 0.7956) (19.9839, 0.7855) (20.0158, 0.7752) (20.0476, 0.7647) (20.0795, 0.7541) (20.1114, 0.7433) (20.1432, 0.7324) (20.175, 0.7213) (20.2068, 0.71) (20.2386, 0.6986) (20.2704, 0.687) (20.3022, 0.6753) (20.3339, 0.6634) (20.3656, 0.6513) (20.3974, 0.6392) (20.4291, 0.6268) (20.4607, 0.6143) (20.4924, 0.6017) (20.5241, 0.5889) (20.5557, 0.576) (20.5873, 0.5629) (20.6189, 0.5497) (20.6505, 0.5364) (20.682, 0.5229) (20.7136, 0.5092) (20.7451, 0.4955) (20.7766, 0.4815) (20.8081, 0.4675) (20.8396, 0.4533) (20.871, 0.439) (20.9024, 0.4245) (20.9338, 0.4099) (20.9589, 0.3982) (20.9777, 0.3893) (20.9903, 0.3833) (20.9966, 0.3803) knots 0 0 0 0 0 0 0.01428571 0.02857143 0.04285714 0.05714286 0.07142857 0.08571429 0.1 0.11428571 0.12857143 0.14285714 0.15714286 0.17142857 0.18571429 0.2 0.21428571 0.22857143 0.24285714 0.25714286 0.27142857 0.28571429 0.3 0.31428571 0.32857143 0.34285714 0.35714286 0.37142857 0.38571429 0.4 0.41428571 0.42857143 0.44285714 0.45714286 0.47142857 0.48571429 0.5 0.51428571 0.52857143 0.54285714 0.55714286 0.57142857 0.58571429 0.6 0.61428571 0.62857143 0.64285714 0.65714286 0.67142857 0.68571429 0.7 0.71428571 0.72857143 0.74285714 0.75714286 0.77142857 0.78571429 0.8 0.81428571 0.82857143 0.84285714 0.85714286 0.87142857 0.88571429 0.9 0.91428571 0.92857143 0.94285714 0.95714286 0.97142857 0.98571429 1 1 1 1 1 1
  arc A0 (20.9966, -0.3803) -> (20.9966, 0.3803) centre (0, 0) ccw
  line L0 (18.7663, 1.0176) -> (18.7663, -1.0176)
  point P0 (18.9244, -1.0125)
  point P1 (19.083, -0.9959)
  point P2 (19.2421, -0.9717)
  point P3 (19.4014, -0.9411)
  point P4 (19.5608, -0.9049)
  point P5 (19.7204, -0.8637)
  point P6 (19.8801, -0.8177)
  point P7 (20.0398, -0.7673)
  point P8 (20.1995, -0.7126)
  point P9 (20.3592, -0.6538)
  point P10 (20.5187, -0.591)
  point P11 (20.6782, -0.5245)
  point P12 (20.8375, -0.4542)
  point P13 (18.9244, 1.0125)
  point P14 (19.083, 0.9959)
  point P15 (19.2421, 0.9717)
  point P16 (19.4014, 0.9411)
  point P17 (19.5608, 0.9049)
  point P18 (19.7204, 0.8637)
  point P19 (19.8801, 0.8177)
  point P20 (20.0398, 0.7673)
  point P21 (20.1995, 0.7126)
  point P22 (20.3592, 0.6538)
  point P23 (20.5187, 0.591)
  point P24 (20.6782, 0.5245)
  point P25 (20.8375, 0.4542)
sketch "Diametrial Pitch Circle" plane through (0, 0, 0) normal (0, 0, 1) x (1, 0, 0)
sketch "Base Circle (1)" plane through (0, 0, 0) normal (0, 0, 1) x (1, 0, 0)
  circle A0 centre (0, 0) radius 28.843
  circle A1 centre (0, 0) radius 2
sketch "Gear Tooth (1)" plane through (0, 0, 0) normal (0, 0, 1) x (1, 0, 0)
  spline S0 degree 5 poles (28.167, -1.1579) (28.1751, -1.1579) (28.1914, -1.1578) (28.2159, -1.1575) (28.2485, -1.1567) (28.2892, -1.1551) (28.33, -1.1529) (28.3707, -1.1501) (28.4115, -1.1467) (28.4523, -1.1427) (28.493, -1.1383) (28.5338, -1.1335) (28.5746, -1.1284) (28.6154, -1.1228) (28.6561, -1.117) (28.6969, -1.1109) (28.7376, -1.1045) (28.7783, -1.0977) (28.8191, -1.0907) (28.8598, -1.0834) (28.9005, -1.0758) (28.9412, -1.0679) (28.9819, -1.0597) (29.0226, -1.0513) (29.0633, -1.0427) (29.104, -1.0338) (29.1446, -1.0247) (29.1853, -1.0153) (29.2259, -1.0057) (29.2665, -0.9959) (29.3071, -0.9858) (29.3477, -0.9755) (29.3883, -0.965) (29.4289, -0.9543) (29.4694, -0.9434) (29.5099, -0.9323) (29.5505, -0.921) (29.591, -0.9094) (29.6315, -0.8977) (29.672, -0.8858) (29.7124, -0.8737) (29.7529, -0.8614) (29.7933, -0.8488) (29.8337, -0.8361) (29.8741, -0.8233) (29.9145, -0.8102) (29.9549, -0.7969) (29.9952, -0.7835) (30.0355, -0.7699) (30.0759, -0.7561) (30.1161, -0.7421) (30.1564, -0.728) (30.1967, -0.7137) (30.2369, -0.6992) (30.2771, -0.6845) (30.3173, -0.6697) (30.3575, -0.6547) (30.3977, -0.6396) (30.4378, -0.6242) (30.4779, -0.6087) (30.518, -0.5931) (30.5581, -0.5773) (30.5982, -0.5613) (30.6382, -0.5451) (30.6782, -0.5288) (30.7182, -0.5124) (30.7582, -0.4958) (30.7981, -0.479) (30.838, -0.4621) (30.8779, -0.445) (30.9178, -0.4278) (30.9497, -0.4139) (30.9736, -0.4034) (30.9895, -0.3963) (30.9975, -0.3928) knots 0 0 0 0 0 0 0.01428571 0.02857143 0.04285714 0.05714286 0.07142857 0.08571429 0.1 0.11428571 0.12857143 0.14285714 0.15714286 0.17142857 0.18571429 0.2 0.21428571 0.22857143 0.24285714 0.25714286 0.27142857 0.28571429 0.3 0.31428571 0.32857143 0.34285714 0.35714286 0.37142857 0.38571429 0.4 0.41428571 0.42857143 0.44285714 0.45714286 0.47142857 0.48571429 0.5 0.51428571 0.52857143 0.54285714 0.55714286 0.57142857 0.58571429 0.6 0.61428571 0.62857143 0.64285714 0.65714286 0.67142857 0.68571429 0.7 0.71428571 0.72857143 0.74285714 0.75714286 0.77142857 0.78571429 0.8 0.81428571 0.82857143 0.84285714 0.85714286 0.87142857 0.88571429 0.9 0.91428571 0.92857143 0.94285714 0.95714286 0.97142857 0.98571429 1 1 1 1 1 1
  spline S1 degree 5 poles (28.167, 1.1579) (28.1751, 1.1579) (28.1914, 1.1578) (28.2159, 1.1575) (28.2485, 1.1567) (28.2892, 1.1551) (28.33, 1.1529) (28.3707, 1.1501) (28.4115, 1.1467) (28.4523, 1.1427) (28.493, 1.1383) (28.5338, 1.1335) (28.5746, 1.1284) (28.6154, 1.1228) (28.6561, 1.117) (28.6969, 1.1109) (28.7376, 1.1045) (28.7783, 1.0977) (28.8191, 1.0907) (28.8598, 1.0834) (28.9005, 1.0758) (28.9412, 1.0679) (28.9819, 1.0597) (29.0226, 1.0513) (29.0633, 1.0427) (29.104, 1.0338) (29.1446, 1.0247) (29.1853, 1.0153) (29.2259, 1.0057) (29.2665, 0.9959) (29.3071, 0.9858) (29.3477, 0.9755) (29.3883, 0.965) (29.4289, 0.9543) (29.4694, 0.9434) (29.5099, 0.9323) (29.5505, 0.921) (29.591, 0.9094) (29.6315, 0.8977) (29.672, 0.8858) (29.7124, 0.8737) (29.7529, 0.8614) (29.7933, 0.8488) (29.8337, 0.8361) (29.8741, 0.8233) (29.9145, 0.8102) (29.9549, 0.7969) (29.9952, 0.7835) (30.0355, 0.7699) (30.0759, 0.7561) (30.1161, 0.7421) (30.1564, 0.728) (30.1967, 0.7137) (30.2369, 0.6992) (30.2771, 0.6845) (30.3173, 0.6697) (30.3575, 0.6547) (30.3977, 0.6396) (30.4378, 0.6242) (30.4779, 0.6087) (30.518, 0.5931) (30.5581, 0.5773) (30.5982, 0.5613) (30.6382, 0.5451) (30.6782, 0.5288) (30.7182, 0.5124) (30.7582, 0.4958) (30.7981, 0.479) (30.838, 0.4621) (30.8779, 0.445) (30.9178, 0.4278) (30.9497, 0.4139) (30.9736, 0.4034) (30.9895, 0.3963) (30.9975, 0.3928) knots 0 0 0 0 0 0 0.01428571 0.02857143 0.04285714 0.05714286 0.07142857 0.08571429 0.1 0.11428571 0.12857143 0.14285714 0.15714286 0.17142857 0.18571429 0.2 0.21428571 0.22857143 0.24285714 0.25714286 0.27142857 0.28571429 0.3 0.31428571 0.32857143 0.34285714 0.35714286 0.37142857 0.38571429 0.4 0.41428571 0.42857143 0.44285714 0.45714286 0.47142857 0.48571429 0.5 0.51428571 0.52857143 0.54285714 0.55714286 0.57142857 0.58571429 0.6 0.61428571 0.62857143 0.64285714 0.65714286 0.67142857 0.68571429 0.7 0.71428571 0.72857143 0.74285714 0.75714286 0.77142857 0.78571429 0.8 0.81428571 0.82857143 0.84285714 0.85714286 0.87142857 0.88571429 0.9 0.91428571 0.92857143 0.94285714 0.95714286 0.97142857 0.98571429 1 1 1 1 1 1
  arc A0 (30.9975, -0.3928) -> (30.9975, 0.3928) centre (0, 0) ccw
  line L0 (28.167, 1.1579) -> (28.167, -1.1579)
  point P0 (28.3681, -1.1501)
  point P1 (28.5698, -1.1289)
  point P2 (28.7718, -1.0988)
  point P3 (28.974, -1.0613)
  point P4 (29.1763, -1.0173)
  point P5 (29.3788, -0.9675)
  point P6 (29.5813, -0.9122)
  point P7 (29.7839, -0.8517)
  point P8 (29.9864, -0.7864)
  point P9 (30.1889, -0.7164)
  point P10 (30.3912, -0.6419)
  point P11 (30.5935, -0.5631)
  point P12 (30.7956, -0.48)
  point P13 (28.3681, 1.1501)
  point P14 (28.5698, 1.1289)
  point P15 (28.7718, 1.0988)
  point P16 (28.974, 1.0613)
  point P17 (29.1763, 1.0173)
  point P18 (29.3788, 0.9675)
  point P19 (29.5813, 0.9122)
  point P20 (29.7839, 0.8517)
  point P21 (29.9864, 0.7864)
  point P22 (30.1889, 0.7164)
  point P23 (30.3912, 0.6419)
  point P24 (30.5935, 0.5631)
  point P25 (30.7956, 0.48)
sketch "Diametrial Pitch Circle (1)" plane through (0, 0, 0) normal (0, 0, 1) x (1, 0, 0)